Autodesk Fusion 360 part; units mm, degrees
(part 12 of 14)
  line L8266 (240.2049, 412.75) -> (245.7042, 403.225)
  line L8267 (245.7042, 403.225) -> (256.7027, 403.225)
  line L8268 (262.202, 412.75) -> (256.7027, 422.275)
  line L8269 (256.7027, 403.225) -> (262.202, 412.75)
  line L8270 (275.9501, 433.3875) -> (264.9516, 433.3875)
  line L8271 (264.9516, 433.3875) -> (259.4524, 423.8625)
  line L8272 (259.4524, 423.8625) -> (264.9516, 414.3375)
  line L8273 (264.9516, 414.3375) -> (275.9501, 414.3375)
  line L8274 (281.4494, 423.8625) -> (275.9501, 433.3875)
  line L8275 (275.9501, 414.3375) -> (281.4494, 423.8625)
  line L8276 (295.1976, 444.5) -> (284.199, 444.5)
  line L8277 (284.199, 444.5) -> (278.6998, 434.975)
  line L8278 (278.6998, 434.975) -> (284.199, 425.45)
  line L8279 (284.199, 425.45) -> (295.1976, 425.45)
  line L8280 (300.6968, 434.975) -> (295.1976, 444.5)
  line L8281 (295.1976, 425.45) -> (300.6968, 434.975)
  line L8282 (314.445, 455.6125) -> (303.4464, 455.6125)
  line L8283 (303.4464, 455.6125) -> (297.9472, 446.0875)
  line L8284 (297.9472, 446.0875) -> (303.4464, 436.5625)
  line L8285 (303.4464, 436.5625) -> (314.445, 436.5625)
  line L8286 (319.9442, 446.0875) -> (314.445, 455.6125)
  line L8287 (314.445, 436.5625) -> (319.9442, 446.0875)
  line L8288 (333.6924, 466.725) -> (322.6939, 466.725)
  line L8289 (322.6939, 466.725) -> (317.1946, 457.2)
  line L8290 (317.1946, 457.2) -> (322.6939, 447.675)
  line L8291 (322.6939, 447.675) -> (333.6924, 447.675)
  line L8292 (339.1916, 457.2) -> (333.6924, 466.725)
  line L8293 (333.6924, 447.675) -> (339.1916, 457.2)
  line L8294 (-821.1525, -177.8) -> (-832.151, -177.8)
  line L8295 (-832.151, -177.8) -> (-837.6503, -187.325)
  line L8296 (-837.6503, -187.325) -> (-832.151, -196.85)
  line L8297 (-832.151, -196.85) -> (-821.1525, -196.85)
  line L8298 (-815.6532, -187.325) -> (-821.1525, -177.8)
  line L8299 (-821.1525, -196.85) -> (-815.6532, -187.325)
  line L8300 (-801.9051, -166.6875) -> (-812.9036, -166.6875)
  line L8301 (-812.9036, -166.6875) -> (-818.4029, -176.2125)
  line L8302 (-818.4029, -176.2125) -> (-812.9036, -185.7375)
  line L8303 (-812.9036, -185.7375) -> (-801.9051, -185.7375)
  line L8304 (-796.4058, -176.2125) -> (-801.9051, -166.6875)
  line L8305 (-801.9051, -185.7375) -> (-796.4058, -176.2125)
  line L8306 (-782.6577, -155.575) -> (-793.6562, -155.575)
  line L8307 (-793.6562, -155.575) -> (-799.1554, -165.1)
  line L8308 (-799.1554, -165.1) -> (-793.6562, -174.625)
  line L8309 (-793.6562, -174.625) -> (-782.6577, -174.625)
  line L8310 (-777.1584, -165.1) -> (-782.6577, -155.575)
  line L8311 (-782.6577, -174.625) -> (-777.1584, -165.1)
  line L8312 (-763.4102, -144.4625) -> (-774.4088, -144.4625)
  line L8313 (-774.4088, -144.4625) -> (-779.908, -153.9875)
  line L8314 (-779.908, -153.9875) -> (-774.4088, -163.5125)
  line L8315 (-774.4088, -163.5125) -> (-763.4102, -163.5125)
  line L8316 (-757.911, -153.9875) -> (-763.4102, -144.4625)
  line L8317 (-763.4102, -163.5125) -> (-757.911, -153.9875)
  line L8318 (-744.1628, -133.35) -> (-755.1614, -133.35)
  line L8319 (-755.1614, -133.35) -> (-760.6606, -142.875)
  line L8320 (-760.6606, -142.875) -> (-755.1614, -152.4)
  line L8321 (-755.1614, -152.4) -> (-744.1628, -152.4)
  line L8322 (-738.6636, -142.875) -> (-744.1628, -133.35)
  line L8323 (-744.1628, -152.4) -> (-738.6636, -142.875)
  line L8324 (-724.9154, -122.2375) -> (-735.9139, -122.2375)
  line L8325 (-735.9139, -122.2375) -> (-741.4132, -131.7625)
  line L8326 (-741.4132, -131.7625) -> (-735.9139, -141.2875)
  line L8327 (-735.9139, -141.2875) -> (-724.9154, -141.2875)
  line L8328 (-719.4162, -131.7625) -> (-724.9154, -122.2375)
  line L8329 (-724.9154, -141.2875) -> (-719.4162, -131.7625)
  line L8330 (-705.668, -111.125) -> (-716.6665, -111.125)
  line L8331 (-716.6665, -111.125) -> (-722.1658, -120.65)
  line L8332 (-722.1658, -120.65) -> (-716.6665, -130.175)
  line L8333 (-716.6665, -130.175) -> (-705.668, -130.175)
  line L8334 (-700.1687, -120.65) -> (-705.668, -111.125)
  line L8335 (-705.668, -130.175) -> (-700.1687, -120.65)
  line L8336 (-686.4206, -100.0125) -> (-697.4191, -100.0125)
  line L8337 (-697.4191, -100.0125) -> (-702.9184, -109.5375)
  line L8338 (-702.9184, -109.5375) -> (-697.4191, -119.0625)
  line L8339 (-697.4191, -119.0625) -> (-686.4206, -119.0625)
  line L8340 (-680.9213, -109.5375) -> (-686.4206, -100.0125)
  line L8341 (-686.4206, -119.0625) -> (-680.9213, -109.5375)
  line L8342 (-667.1732, -88.9) -> (-678.1717, -88.9)
  line L8343 (-678.1717, -88.9) -> (-683.671, -98.425)
  line L8344 (-683.671, -98.425) -> (-678.1717, -107.95)
  line L8345 (-678.1717, -107.95) -> (-667.1732, -107.95)
  line L8346 (-661.6739, -98.425) -> (-667.1732, -88.9)
  line L8347 (-667.1732, -107.95) -> (-661.6739, -98.425)
  line L8348 (-647.9258, -77.7875) -> (-658.9243, -77.7875)
  line L8349 (-658.9243, -77.7875) -> (-664.4235, -87.3125)
  line L8350 (-664.4235, -87.3125) -> (-658.9243, -96.8375)
  line L8351 (-658.9243, -96.8375) -> (-647.9258, -96.8375)
  line L8352 (-642.4265, -87.3125) -> (-647.9258, -77.7875)
  line L8353 (-647.9258, -96.8375) -> (-642.4265, -87.3125)
  line L8354 (-628.6783, -66.675) -> (-639.6769, -66.675)
  line L8355 (-639.6769, -66.675) -> (-645.1761, -76.2)
  line L8356 (-645.1761, -76.2) -> (-639.6769, -85.725)
  line L8357 (-639.6769, -85.725) -> (-628.6783, -85.725)
  line L8358 (-623.1791, -76.2) -> (-628.6783, -66.675)
  line L8359 (-628.6783, -85.725) -> (-623.1791, -76.2)
  line L8360 (-609.4309, -55.5625) -> (-620.4295, -55.5625)
  line L8361 (-620.4295, -55.5625) -> (-625.9287, -65.0875)
  line L8362 (-625.9287, -65.0875) -> (-620.4295, -74.6125)
  line L8363 (-620.4295, -74.6125) -> (-609.4309, -74.6125)
  line L8364 (-603.9317, -65.0875) -> (-609.4309, -55.5625)
  line L8365 (-609.4309, -74.6125) -> (-603.9317, -65.0875)
  line L8366 (-590.1835, -44.45) -> (-601.182, -44.45)
  line L8367 (-601.182, -44.45) -> (-606.6813, -53.975)
  line L8368 (-606.6813, -53.975) -> (-601.182, -63.5)
  line L8369 (-601.182, -63.5) -> (-590.1835, -63.5)
  line L8370 (-584.6843, -53.975) -> (-590.1835, -44.45)
  line L8371 (-590.1835, -63.5) -> (-584.6843, -53.975)
  line L8372 (-570.9361, -33.3375) -> (-581.9346, -33.3375)
  line L8373 (-581.9346, -33.3375) -> (-587.4339, -42.8625)
  line L8374 (-587.4339, -42.8625) -> (-581.9346, -52.3875)
  line L8375 (-581.9346, -52.3875) -> (-570.9361, -52.3875)
  line L8376 (-565.4368, -42.8625) -> (-570.9361, -33.3375)
  line L8377 (-570.9361, -52.3875) -> (-565.4368, -42.8625)
  line L8378 (-551.6887, -22.225) -> (-562.6872, -22.225)
  line L8379 (-562.6872, -22.225) -> (-568.1865, -31.75)
  line L8380 (-568.1865, -31.75) -> (-562.6872, -41.275)
  line L8381 (-562.6872, -41.275) -> (-551.6887, -41.275)
  line L8382 (-546.1894, -31.75) -> (-551.6887, -22.225)
  line L8383 (-551.6887, -41.275) -> (-546.1894, -31.75)
  line L8384 (-532.4413, -11.1125) -> (-543.4398, -11.1125)
  line L8385 (-543.4398, -11.1125) -> (-548.9391, -20.6375)
  line L8386 (-548.9391, -20.6375) -> (-543.4398, -30.1625)
  line L8387 (-543.4398, -30.1625) -> (-532.4413, -30.1625)
  line L8388 (-526.942, -20.6375) -> (-532.4413, -11.1125)
  line L8389 (-532.4413, -30.1625) -> (-526.942, -20.6375)
  line L8390 (-513.1939, 0) -> (-524.1924, 0)
  line L8391 (-524.1924, 0) -> (-529.6916, -9.525)
  line L8392 (-529.6916, -9.525) -> (-524.1924, -19.05)
  line L8393 (-524.1924, -19.05) -> (-513.1939, -19.05)
  line L8394 (-507.6946, -9.525) -> (-513.1939, 0)
  line L8395 (-513.1939, -19.05) -> (-507.6946, -9.525)
  line L8396 (-493.9464, 11.1125) -> (-504.945, 11.1125)
  line L8397 (-504.945, 11.1125) -> (-510.4442, 1.5875)
  line L8398 (-510.4442, 1.5875) -> (-504.945, -7.9375)
  line L8399 (-504.945, -7.9375) -> (-493.9464, -7.9375)
  line L8400 (-488.4472, 1.5875) -> (-493.9464, 11.1125)
  line L8401 (-493.9464, -7.9375) -> (-488.4472, 1.5875)
  line L8402 (-474.699, 22.225) -> (-485.6976, 22.225)
  line L8403 (-485.6976, 22.225) -> (-491.1968, 12.7)
  line L8404 (-491.1968, 12.7) -> (-485.6976, 3.175)
  line L8405 (-485.6976, 3.175) -> (-474.699, 3.175)
  line L8406 (-469.1998, 12.7) -> (-474.699, 22.225)
  line L8407 (-474.699, 3.175) -> (-469.1998, 12.7)
  line L8408 (-455.4516, 33.3375) -> (-466.4501, 33.3375)
  line L8409 (-466.4501, 33.3375) -> (-471.9494, 23.8125)
  line L8410 (-471.9494, 23.8125) -> (-466.4501, 14.2875)
  line L8411 (-466.4501, 14.2875) -> (-455.4516, 14.2875)
  line L8412 (-449.9524, 23.8125) -> (-455.4516, 33.3375)
  line L8413 (-455.4516, 14.2875) -> (-449.9524, 23.8125)
  line L8414 (-436.2042, 44.45) -> (-447.2027, 44.45)
  line L8415 (-447.2027, 44.45) -> (-452.702, 34.925)
  line L8416 (-452.702, 34.925) -> (-447.2027, 25.4)
  line L8417 (-447.2027, 25.4) -> (-436.2042, 25.4)
  line L8418 (-430.7049, 34.925) -> (-436.2042, 44.45)
  line L8419 (-436.2042, 25.4) -> (-430.7049, 34.925)
  line L8420 (-416.9568, 55.5625) -> (-427.9553, 55.5625)
  line L8421 (-427.9553, 55.5625) -> (-433.4546, 46.0375)
  line L8422 (-433.4546, 46.0375) -> (-427.9553, 36.5125)
  line L8423 (-427.9553, 36.5125) -> (-416.9568, 36.5125)
  line L8424 (-411.4575, 46.0375) -> (-416.9568, 55.5625)
  line L8425 (-416.9568, 36.5125) -> (-411.4575, 46.0375)
  line L8426 (-397.7094, 66.675) -> (-408.7079, 66.675)
  line L8427 (-408.7079, 66.675) -> (-414.2072, 57.15)
  line L8428 (-414.2072, 57.15) -> (-408.7079, 47.625)
  line L8429 (-408.7079, 47.625) -> (-397.7094, 47.625)
  line L8430 (-392.2101, 57.15) -> (-397.7094, 66.675)
  line L8431 (-397.7094, 47.625) -> (-392.2101, 57.15)
  line L8432 (-378.462, 77.7875) -> (-389.4605, 77.7875)
  line L8433 (-389.4605, 77.7875) -> (-394.9597, 68.2625)
  line L8434 (-394.9597, 68.2625) -> (-389.4605, 58.7375)
  line L8435 (-389.4605, 58.7375) -> (-378.462, 58.7375)
  line L8436 (-372.9627, 68.2625) -> (-378.462, 77.7875)
  line L8437 (-378.462, 58.7375) -> (-372.9627, 68.2625)
  line L8438 (-359.2145, 88.9) -> (-370.2131, 88.9)
  line L8439 (-370.2131, 88.9) -> (-375.7123, 79.375)
  line L8440 (-375.7123, 79.375) -> (-370.2131, 69.85)
  line L8441 (-370.2131, 69.85) -> (-359.2145, 69.85)
  line L8442 (-353.7153, 79.375) -> (-359.2145, 88.9)
  line L8443 (-359.2145, 69.85) -> (-353.7153, 79.375)
  line L8444 (-339.9671, 100.0125) -> (-350.9657, 100.0125)
  line L8445 (-350.9657, 100.0125) -> (-356.4649, 90.4875)
  line L8446 (-356.4649, 90.4875) -> (-350.9657, 80.9625)
  line L8447 (-350.9657, 80.9625) -> (-339.9671, 80.9625)
  line L8448 (-334.4679, 90.4875) -> (-339.9671, 100.0125)
  line L8449 (-339.9671, 80.9625) -> (-334.4679, 90.4875)
  line L8450 (-320.7197, 111.125) -> (-331.7182, 111.125)
  line L8451 (-331.7182, 111.125) -> (-337.2175, 101.6)
  line L8452 (-337.2175, 101.6) -> (-331.7182, 92.075)
  line L8453 (-331.7182, 92.075) -> (-320.7197, 92.075)
  line L8454 (-315.2205, 101.6) -> (-320.7197, 111.125)
  line L8455 (-320.7197, 92.075) -> (-315.2205, 101.6)
  line L8456 (-301.4723, 122.2375) -> (-312.4708, 122.2375)
  line L8457 (-312.4708, 122.2375) -> (-317.9701, 112.7125)
  line L8458 (-317.9701, 112.7125) -> (-312.4708, 103.1875)
  line L8459 (-312.4708, 103.1875) -> (-301.4723, 103.1875)
  line L8460 (-295.973, 112.7125) -> (-301.4723, 122.2375)
  line L8461 (-301.4723, 103.1875) -> (-295.973, 112.7125)
  line L8462 (-282.2249, 133.35) -> (-293.2234, 133.35)
  line L8463 (-293.2234, 133.35) -> (-298.7227, 123.825)
  line L8464 (-298.7227, 123.825) -> (-293.2234, 114.3)
  line L8465 (-293.2234, 114.3) -> (-282.2249, 114.3)
  line L8466 (-276.7256, 123.825) -> (-282.2249, 133.35)
  line L8467 (-282.2249, 114.3) -> (-276.7256, 123.825)
  line L8468 (-262.9775, 144.4625) -> (-273.976, 144.4625)
  line L8469 (-273.976, 144.4625) -> (-279.4753, 134.9375)
  line L8470 (-279.4753, 134.9375) -> (-273.976, 125.4125)
  line L8471 (-273.976, 125.4125) -> (-262.9775, 125.4125)
  line L8472 (-257.4782, 134.9375) -> (-262.9775, 144.4625)
  line L8473 (-262.9775, 125.4125) -> (-257.4782, 134.9375)
  line L8474 (-243.7301, 155.575) -> (-254.7286, 155.575)
  line L8475 (-254.7286, 155.575) -> (-260.2278, 146.05)
  line L8476 (-260.2278, 146.05) -> (-254.7286, 136.525)
  line L8477 (-254.7286, 136.525) -> (-243.7301, 136.525)
  line L8478 (-238.2308, 146.05) -> (-243.7301, 155.575)
  line L8479 (-243.7301, 136.525) -> (-238.2308, 146.05)
  line L8480 (-224.4826, 166.6875) -> (-235.4812, 166.6875)
  line L8481 (-235.4812, 166.6875) -> (-240.9804, 157.1625)
  line L8482 (-240.9804, 157.1625) -> (-235.4812, 147.6375)
  line L8483 (-235.4812, 147.6375) -> (-224.4826, 147.6375)
  line L8484 (-218.9834, 157.1625) -> (-224.4826, 166.6875)
  line L8485 (-224.4826, 147.6375) -> (-218.9834, 157.1625)
  line L8486 (-205.2352, 177.8) -> (-216.2337, 177.8)
  line L8487 (-216.2337, 177.8) -> (-221.733, 168.275)
  line L8488 (-221.733, 168.275) -> (-216.2337, 158.75)
  line L8489 (-216.2337, 158.75) -> (-205.2352, 158.75)
  line L8490 (-199.736, 168.275) -> (-205.2352, 177.8)
  line L8491 (-205.2352, 158.75) -> (-199.736, 168.275)
  line L8492 (-185.9878, 188.9125) -> (-196.9863, 188.9125)
  line L8493 (-196.9863, 188.9125) -> (-202.4856, 179.3875)
  line L8494 (-202.4856, 179.3875) -> (-196.9863, 169.8625)
  line L8495 (-196.9863, 169.8625) -> (-185.9878, 169.8625)
  line L8496 (-180.4886, 179.3875) -> (-185.9878, 188.9125)
  line L8497 (-185.9878, 169.8625) -> (-180.4886, 179.3875)
  line L8498 (-166.7404, 200.025) -> (-177.7389, 200.025)
  line L8499 (-177.7389, 200.025) -> (-183.2382, 190.5)
  line L8500 (-183.2382, 190.5) -> (-177.7389, 180.975)
  line L8501 (-177.7389, 180.975) -> (-166.7404, 180.975)
  line L8502 (-161.2411, 190.5) -> (-166.7404, 200.025)
  line L8503 (-166.7404, 180.975) -> (-161.2411, 190.5)
  line L8504 (-147.493, 211.1375) -> (-158.4915, 211.1375)
  line L8505 (-158.4915, 211.1375) -> (-163.9908, 201.6125)
  line L8506 (-163.9908, 201.6125) -> (-158.4915, 192.0875)
  line L8507 (-158.4915, 192.0875) -> (-147.493, 192.0875)
  line L8508 (-141.9937, 201.6125) -> (-147.493, 211.1375)
  line L8509 (-147.493, 192.0875) -> (-141.9937, 201.6125)
  line L8510 (-128.2456, 222.25) -> (-139.2441, 222.25)
  line L8511 (-139.2441, 222.25) -> (-144.7434, 212.725)
  line L8512 (-144.7434, 212.725) -> (-139.2441, 203.2)
  line L8513 (-139.2441, 203.2) -> (-128.2456, 203.2)
  line L8514 (-122.7463, 212.725) -> (-128.2456, 222.25)
  line L8515 (-128.2456, 203.2) -> (-122.7463, 212.725)
  line L8516 (-108.9982, 233.3625) -> (-119.9967, 233.3625)
  line L8517 (-119.9967, 233.3625) -> (-125.4959, 223.8375)
  line L8518 (-125.4959, 223.8375) -> (-119.9967, 214.3125)
  line L8519 (-119.9967, 214.3125) -> (-108.9982, 214.3125)
  line L8520 (-103.4989, 223.8375) -> (-108.9982, 233.3625)
  line L8521 (-108.9982, 214.3125) -> (-103.4989, 223.8375)
  line L8522 (-89.7507, 244.475) -> (-100.7493, 244.475)
  line L8523 (-100.7493, 244.475) -> (-106.2485, 234.95)
  line L8524 (-106.2485, 234.95) -> (-100.7493, 225.425)
  line L8525 (-100.7493, 225.425) -> (-89.7507, 225.425)
  line L8526 (-84.2515, 234.95) -> (-89.7507, 244.475)
  line L8527 (-89.7507, 225.425) -> (-84.2515, 234.95)
  line L8528 (-70.5033, 255.5875) -> (-81.5018, 255.5875)
  line L8529 (-81.5018, 255.5875) -> (-87.0011, 246.0625)
  line L8530 (-87.0011, 246.0625) -> (-81.5018, 236.5375)
  line L8531 (-81.5018, 236.5375) -> (-70.5033, 236.5375)
  line L8532 (-65.0041, 246.0625) -> (-70.5033, 255.5875)
  line L8533 (-70.5033, 236.5375) -> (-65.0041, 246.0625)
  line L8534 (-51.2559, 266.7) -> (-62.2544, 266.7)
  line L8535 (-62.2544, 266.7) -> (-67.7537, 257.175)
  line L8536 (-67.7537, 257.175) -> (-62.2544, 247.65)
  line L8537 (-62.2544, 247.65) -> (-51.2559, 247.65)
  line L8538 (-45.7566, 257.175) -> (-51.2559, 266.7)
  line L8539 (-51.2559, 247.65) -> (-45.7566, 257.175)
  line L8540 (-32.0085, 277.8125) -> (-43.007, 277.8125)
  line L8541 (-43.007, 277.8125) -> (-48.5063, 268.2875)
  line L8542 (-48.5063, 268.2875) -> (-43.007, 258.7625)
  line L8543 (-43.007, 258.7625) -> (-32.0085, 258.7625)
  line L8544 (-26.5092, 268.2875) -> (-32.0085, 277.8125)
  line L8545 (-32.0085, 258.7625) -> (-26.5092, 268.2875)
  line L8546 (-12.7611, 288.925) -> (-23.7596, 288.925)
  line L8547 (-23.7596, 288.925) -> (-29.2589, 279.4)
  line L8548 (-29.2589, 279.4) -> (-23.7596, 269.875)
  line L8549 (-23.7596, 269.875) -> (-12.7611, 269.875)
  line L8550 (-7.2618, 279.4) -> (-12.7611, 288.925)
  line L8551 (-12.7611, 269.875) -> (-7.2618, 279.4)
  line L8552 (6.4863, 300.0375) -> (-4.5122, 300.0375)
  line L8553 (-4.5122, 300.0375) -> (-10.0114, 290.5125)
  line L8554 (-10.0114, 290.5125) -> (-4.5122, 280.9875)
  line L8555 (-4.5122, 280.9875) -> (6.4863, 280.9875)
  line L8556 (11.9856, 290.5125) -> (6.4863, 300.0375)
  line L8557 (6.4863, 280.9875) -> (11.9856, 290.5125)
  line L8558 (25.7337, 311.15) -> (14.7352, 311.15)
  line L8559 (14.7352, 311.15) -> (9.236, 301.625)
  line L8560 (9.236, 301.625) -> (14.7352, 292.1)
  line L8561 (14.7352, 292.1) -> (25.7337, 292.1)
  line L8562 (31.233, 301.625) -> (25.7337, 311.15)
  line L8563 (25.7337, 292.1) -> (31.233, 301.625)
  line L8564 (44.9812, 322.2625) -> (33.9826, 322.2625)
  line L8565 (33.9826, 322.2625) -> (28.4834, 312.7375)
  line L8566 (28.4834, 312.7375) -> (33.9826, 303.2125)
  line L8567 (33.9826, 303.2125) -> (44.9812, 303.2125)
  line L8568 (50.4804, 312.7375) -> (44.9812, 322.2625)
  line L8569 (44.9812, 303.2125) -> (50.4804, 312.7375)
  line L8570 (64.2286, 333.375) -> (53.2301, 333.375)
  line L8571 (53.2301, 333.375) -> (47.7308, 323.85)
  line L8572 (47.7308, 323.85) -> (53.2301, 314.325)
  line L8573 (53.2301, 314.325) -> (64.2286, 314.325)
  line L8574 (69.7278, 323.85) -> (64.2286, 333.375)
  line L8575 (64.2286, 314.325) -> (69.7278, 323.85)
  line L8576 (83.476, 344.4875) -> (72.4775, 344.4875)
  line L8577 (72.4775, 344.4875) -> (66.9782, 334.9625)
  line L8578 (66.9782, 334.9625) -> (72.4775, 325.4375)
  line L8579 (72.4775, 325.4375) -> (83.476, 325.4375)
  line L8580 (88.9753, 334.9625) -> (83.476, 344.4875)
  line L8581 (83.476, 325.4375) -> (88.9753, 334.9625)
  line L8582 (102.7234, 355.6) -> (91.7249, 355.6)
  line L8583 (91.7249, 355.6) -> (86.2256, 346.075)
  line L8584 (86.2256, 346.075) -> (91.7249, 336.55)
  line L8585 (91.7249, 336.55) -> (102.7234, 336.55)
  line L8586 (108.2227, 346.075) -> (102.7234, 355.6)
  line L8587 (102.7234, 336.55) -> (108.2227, 346.075)
  line L8588 (121.9708, 366.7125) -> (110.9723, 366.7125)
  line L8589 (110.9723, 366.7125) -> (105.473, 357.1875)
  line L8590 (105.473, 357.1875) -> (110.9723, 347.6625)
  line L8591 (110.9723, 347.6625) -> (121.9708, 347.6625)
  line L8592 (127.4701, 357.1875) -> (121.9708, 366.7125)
  line L8593 (121.9708, 347.6625) -> (127.4701, 357.1875)
  line L8594 (141.2182, 377.825) -> (130.2197, 377.825)
  line L8595 (130.2197, 377.825) -> (124.7205, 368.3)
  line L8596 (124.7205, 368.3) -> (130.2197, 358.775)
  line L8597 (130.2197, 358.775) -> (141.2182, 358.775)
  line L8598 (146.7175, 368.3) -> (141.2182, 377.825)
  line L8599 (141.2182, 358.775) -> (146.7175, 368.3)
  line L8600 (160.4657, 388.9375) -> (149.4671, 388.9375)
  line L8601 (149.4671, 388.9375) -> (143.9679, 379.4125)
  line L8602 (143.9679, 379.4125) -> (149.4671, 369.8875)
  line L8603 (149.4671, 369.8875) -> (160.4657, 369.8875)
  line L8604 (165.9649, 379.4125) -> (160.4657, 388.9375)
  line L8605 (160.4657, 369.8875) -> (165.9649, 379.4125)
  line L8606 (179.7131, 400.05) -> (168.7145, 400.05)
  line L8607 (168.7145, 400.05) -> (163.2153, 390.525)
  line L8608 (163.2153, 390.525) -> (168.7145, 381)
  line L8609 (168.7145, 381) -> (179.7131, 381)
  line L8610 (185.2123, 390.525) -> (179.7131, 400.05)
  line L8611 (179.7131, 381) -> (185.2123, 390.525)
  line L8612 (198.9605, 411.1625) -> (187.962, 411.1625)
  line L8613 (187.962, 411.1625) -> (182.4627, 401.6375)
  line L8614 (182.4627, 401.6375) -> (187.962, 392.1125)
  line L8615 (187.962, 392.1125) -> (198.9605, 392.1125)
  line L8616 (204.4597, 401.6375) -> (198.9605, 411.1625)
  line L8617 (198.9605, 392.1125) -> (204.4597, 401.6375)
  line L8618 (218.2079, 422.275) -> (207.2094, 422.275)
  line L8619 (207.2094, 422.275) -> (201.7101, 412.75)
  line L8620 (201.7101, 412.75) -> (207.2094, 403.225)
  line L8621 (207.2094, 403.225) -> (218.2079, 403.225)
  line L8622 (223.7072, 412.75) -> (218.2079, 422.275)
  line L8623 (218.2079, 403.225) -> (223.7072, 412.75)
  line L8624 (237.4553, 433.3875) -> (226.4568, 433.3875)
  line L8625 (226.4568, 433.3875) -> (220.9575, 423.8625)
  line L8626 (220.9575, 423.8625) -> (226.4568, 414.3375)
  line L8627 (226.4568, 414.3375) -> (237.4553, 414.3375)
  line L8628 (242.9546, 423.8625) -> (237.4553, 433.3875)
  line L8629 (237.4553, 414.3375) -> (242.9546, 423.8625)
  line L8630 (256.7027, 444.5) -> (245.7042, 444.5)
  line L8631 (245.7042, 444.5) -> (240.2049, 434.975)
  line L8632 (240.2049, 434.975) -> (245.7042, 425.45)
  line L8633 (245.7042, 425.45) -> (256.7027, 425.45)
  line L8634 (262.202, 434.975) -> (256.7027, 444.5)
  line L8635 (256.7027, 425.45) -> (262.202, 434.975)
  line L8636 (275.9501, 455.6125) -> (264.9516, 455.6125)
  line L8637 (264.9516, 455.6125) -> (259.4524, 446.0875)
  line L8638 (259.4524, 446.0875) -> (264.9516, 436.5625)
  line L8639 (264.9516, 436.5625) -> (275.9501, 436.5625)
  line L8640 (281.4494, 446.0875) -> (275.9501, 455.6125)
  line L8641 (275.9501, 436.5625) -> (281.4494, 446.0875)
  line L8642 (295.1976, 466.725) -> (284.199, 466.725)
  line L8643 (284.199, 466.725) -> (278.6998, 457.2)
  line L8644 (278.6998, 457.2) -> (284.199, 447.675)
  line L8645 (284.199, 447.675) -> (295.1976, 447.675)
  line L8646 (300.6968, 457.2) -> (295.1976, 466.725)
  line L8647 (295.1976, 447.675) -> (300.6968, 457.2)
  line L8648 (314.445, 477.8375) -> (303.4464, 477.8375)
  line L8649 (303.4464, 477.8375) -> (297.9472, 468.3125)
  line L8650 (297.9472, 468.3125) -> (303.4464, 458.7875)
  line L8651 (303.4464, 458.7875) -> (314.445, 458.7875)
  line L8652 (319.9442, 468.3125) -> (314.445, 477.8375)
  line L8653 (314.445, 458.7875) -> (319.9442, 468.3125)
  line L8654 (-840.3999, -166.6875) -> (-851.3984, -166.6875)
  line L8655 (-851.3984, -166.6875) -> (-856.8977, -176.2125)
  line L8656 (-856.8977, -176.2125) -> (-851.3984, -185.7375)
  line L8657 (-851.3984, -185.7375) -> (-840.3999, -185.7375)
  line L8658 (-834.9006, -176.2125) -> (-840.3999, -166.6875)
  line L8659 (-840.3999, -185.7375) -> (-834.9006, -176.2125)
  line L8660 (-821.1525, -155.575) -> (-832.151, -155.575)
  line L8661 (-832.151, -155.575) -> (-837.6503, -165.1)
  line L8662 (-837.6503, -165.1) -> (-832.151, -174.625)
  line L8663 (-832.151, -174.625) -> (-821.1525, -174.625)
  line L8664 (-815.6532, -165.1) -> (-821.1525, -155.575)
  line L8665 (-821.1525, -174.625) -> (-815.6532, -165.1)
  line L8666 (-801.9051, -144.4625) -> (-812.9036, -144.4625)
  line L8667 (-812.9036, -144.4625) -> (-818.4029, -153.9875)
  line L8668 (-818.4029, -153.9875) -> (-812.9036, -163.5125)
  line L8669 (-812.9036, -163.5125) -> (-801.9051, -163.5125)
  line L8670 (-796.4058, -153.9875) -> (-801.9051, -144.4625)
  line L8671 (-801.9051, -163.5125) -> (-796.4058, -153.9875)
  line L8672 (-782.6577, -133.35) -> (-793.6562, -133.35)
  line L8673 (-793.6562, -133.35) -> (-799.1554, -142.875)
  line L8674 (-799.1554, -142.875) -> (-793.6562, -152.4)
  line L8675 (-793.6562, -152.4) -> (-782.6577, -152.4)
  line L8676 (-777.1584, -142.875) -> (-782.6577, -133.35)
  line L8677 (-782.6577, -152.4) -> (-777.1584, -142.875)
  line L8678 (-763.4102, -122.2375) -> (-774.4088, -122.2375)
  line L8679 (-774.4088, -122.2375) -> (-779.908, -131.7625)
  line L8680 (-779.908, -131.7625) -> (-774.4088, -141.2875)
  line L8681 (-774.4088, -141.2875) -> (-763.4102, -141.2875)
  line L8682 (-757.911, -131.7625) -> (-763.4102, -122.2375)
  line L8683 (-763.4102, -141.2875) -> (-757.911, -131.7625)
  line L8684 (-744.1628, -111.125) -> (-755.1614, -111.125)
  line L8685 (-755.1614, -111.125) -> (-760.6606, -120.65)
  line L8686 (-760.6606, -120.65) -> (-755.1614, -130.175)
  line L8687 (-755.1614, -130.175) -> (-744.1628, -130.175)
  line L8688 (-738.6636, -120.65) -> (-744.1628, -111.125)
  line L8689 (-744.1628, -130.175) -> (-738.6636, -120.65)
  line L8690 (-724.9154, -100.0125) -> (-735.9139, -100.0125)
  line L8691 (-735.9139, -100.0125) -> (-741.4132, -109.5375)
  line L8692 (-741.4132, -109.5375) -> (-735.9139, -119.0625)
  line L8693 (-735.9139, -119.0625) -> (-724.9154, -119.0625)
  line L8694 (-719.4162, -109.5375) -> (-724.9154, -100.0125)
  line L8695 (-724.9154, -119.0625) -> (-719.4162, -109.5375)
  line L8696 (-705.668, -88.9) -> (-716.6665, -88.9)
  line L8697 (-716.6665, -88.9) -> (-722.1658, -98.425)
  line L8698 (-722.1658, -98.425) -> (-716.6665, -107.95)
  line L8699 (-716.6665, -107.95) -> (-705.668, -107.95)
  line L8700 (-700.1687, -98.425) -> (-705.668, -88.9)
  line L8701 (-705.668, -107.95) -> (-700.1687, -98.425)
  line L8702 (-686.4206, -77.7875) -> (-697.4191, -77.7875)
  line L8703 (-697.4191, -77.7875) -> (-702.9184, -87.3125)
  line L8704 (-702.9184, -87.3125) -> (-697.4191, -96.8375)
  line L8705 (-697.4191, -96.8375) -> (-686.4206, -96.8375)
  line L8706 (-680.9213, -87.3125) -> (-686.4206, -77.7875)
  line L8707 (-686.4206, -96.8375) -> (-680.9213, -87.3125)
  line L8708 (-667.1732, -66.675) -> (-678.1717, -66.675)
  line L8709 (-678.1717, -66.675) -> (-683.671, -76.2)
  line L8710 (-683.671, -76.2) -> (-678.1717, -85.725)
  line L8711 (-678.1717, -85.725) -> (-667.1732, -85.725)
  line L8712 (-661.6739, -76.2) -> (-667.1732, -66.675)
  line L8713 (-667.1732, -85.725) -> (-661.6739, -76.2)
  line L8714 (-647.9258, -55.5625) -> (-658.9243, -55.5625)
  line L8715 (-658.9243, -55.5625) -> (-664.4235, -65.0875)
  line L8716 (-664.4235, -65.0875) -> (-658.9243, -74.6125)
  line L8717 (-658.9243, -74.6125) -> (-647.9258, -74.6125)
  line L8718 (-642.4265, -65.0875) -> (-647.9258, -55.5625)
  line L8719 (-647.9258, -74.6125) -> (-642.4265, -65.0875)
  line L8720 (-628.6783, -44.45) -> (-639.6769, -44.45)
  line L8721 (-639.6769, -44.45) -> (-645.1761, -53.975)
  line L8722 (-645.1761, -53.975) -> (-639.6769, -63.5)
  line L8723 (-639.6769, -63.5) -> (-628.6783, -63.5)
  line L8724 (-623.1791, -53.975) -> (-628.6783, -44.45)
  line L8725 (-628.6783, -63.5) -> (-623.1791, -53.975)
  line L8726 (-609.4309, -33.3375) -> (-620.4295, -33.3375)
  line L8727 (-620.4295, -33.3375) -> (-625.9287, -42.8625)
  line L8728 (-625.9287, -42.8625) -> (-620.4295, -52.3875)
  line L8729 (-620.4295, -52.3875) -> (-609.4309, -52.3875)
  line L8730 (-603.9317, -42.8625) -> (-609.4309, -33.3375)
  line L8731 (-609.4309, -52.3875) -> (-603.9317, -42.8625)
  line L8732 (-590.1835, -22.225) -> (-601.182, -22.225)
  line L8733 (-601.182, -22.225) -> (-606.6813, -31.75)
  line L8734 (-606.6813, -31.75) -> (-601.182, -41.275)
  line L8735 (-601.182, -41.275) -> (-590.1835, -41.275)
  line L8736 (-584.6843, -31.75) -> (-590.1835, -22.225)
  line L8737 (-590.1835, -41.275) -> (-584.6843, -31.75)
  line L8738 (-570.9361, -11.1125) -> (-581.9346, -11.1125)
  line L8739 (-581.9346, -11.1125) -> (-587.4339, -20.6375)
  line L8740 (-587.4339, -20.6375) -> (-581.9346, -30.1625)
  line L8741 (-581.9346, -30.1625) -> (-570.9361, -30.1625)
  line L8742 (-565.4368, -20.6375) -> (-570.9361, -11.1125)
  line L8743 (-570.9361, -30.1625) -> (-565.4368, -20.6375)
  line L8744 (-551.6887, 0) -> (-562.6872, 0)
  line L8745 (-562.6872, 0) -> (-568.1865, -9.525)
  line L8746 (-568.1865, -9.525) -> (-562.6872, -19.05)
  line L8747 (-562.6872, -19.05) -> (-551.6887, -19.05)
  line L8748 (-546.1894, -9.525) -> (-551.6887, 0)
  line L8749 (-551.6887, -19.05) -> (-546.1894, -9.525)
  line L8750 (-532.4413, 11.1125) -> (-543.4398, 11.1125)
  line L8751 (-543.4398, 11.1125) -> (-548.9391, 1.5875)
  line L8752 (-548.9391, 1.5875) -> (-543.4398, -7.9375)
  line L8753 (-543.4398, -7.9375) -> (-532.4413, -7.9375)
  line L8754 (-526.942, 1.5875) -> (-532.4413, 11.1125)
  line L8755 (-532.4413, -7.9375) -> (-526.942, 1.5875)
  line L8756 (-513.1939, 22.225) -> (-524.1924, 22.225)
  line L8757 (-524.1924, 22.225) -> (-529.6916, 12.7)
  line L8758 (-529.6916, 12.7) -> (-524.1924, 3.175)
  line L8759 (-524.1924, 3.175) -> (-513.1939, 3.175)
  line L8760 (-507.6946, 12.7) -> (-513.1939, 22.225)
  line L8761 (-513.1939, 3.175) -> (-507.6946, 12.7)
  line L8762 (-493.9464, 33.3375) -> (-504.945, 33.3375)
  line L8763 (-504.945, 33.3375) -> (-510.4442, 23.8125)
  line L8764 (-510.4442, 23.8125) -> (-504.945, 14.2875)
  line L8765 (-504.945, 14.2875) -> (-493.9464, 14.2875)
  line L8766 (-488.4472, 23.8125) -> (-493.9464, 33.3375)
  line L8767 (-493.9464, 14.2875) -> (-488.4472, 23.8125)
  line L8768 (-474.699, 44.45) -> (-485.6976, 44.45)
  line L8769 (-485.6976, 44.45) -> (-491.1968, 34.925)
  line L8770 (-491.1968, 34.925) -> (-485.6976, 25.4)
  line L8771 (-485.6976, 25.4) -> (-474.699, 25.4)
  line L8772 (-469.1998, 34.925) -> (-474.699, 44.45)
  line L8773 (-474.699, 25.4) -> (-469.1998, 34.925)
  line L8774 (-455.4516, 55.5625) -> (-466.4501, 55.5625)
  line L8775 (-466.4501, 55.5625) -> (-471.9494, 46.0375)
  line L8776 (-471.9494, 46.0375) -> (-466.4501, 36.5125)
  line L8777 (-466.4501, 36.5125) -> (-455.4516, 36.5125)
  line L8778 (-449.9524, 46.0375) -> (-455.4516, 55.5625)
  line L8779 (-455.4516, 36.5125) -> (-449.9524, 46.0375)
  line L8780 (-436.2042, 66.675) -> (-447.2027, 66.675)
  line L8781 (-447.2027, 66.675) -> (-452.702, 57.15)
  line L8782 (-452.702, 57.15) -> (-447.2027, 47.625)
  line L8783 (-447.2027, 47.625) -> (-436.2042, 47.625)
  line L8784 (-430.7049, 57.15) -> (-436.2042, 66.675)
  line L8785 (-436.2042, 47.625) -> (-430.7049, 57.15)
  line L8786 (-416.9568, 77.7875) -> (-427.9553, 77.7875)
  line L8787 (-427.9553, 77.7875) -> (-433.4546, 68.2625)
  line L8788 (-433.4546, 68.2625) -> (-427.9553, 58.7375)
  line L8789 (-427.9553, 58.7375) -> (-416.9568, 58.7375)
  line L8790 (-411.4575, 68.2625) -> (-416.9568, 77.7875)
  line L8791 (-416.9568, 58.7375) -> (-411.4575, 68.2625)
  line L8792 (-397.7094, 88.9) -> (-408.7079, 88.9)
  line L8793 (-408.7079, 88.9) -> (-414.2072, 79.375)
  line L8794 (-414.2072, 79.375) -> (-408.7079, 69.85)
  line L8795 (-408.7079, 69.85) -> (-397.7094, 69.85)
  line L8796 (-392.2101, 79.375) -> (-397.7094, 88.9)
  line L8797 (-397.7094, 69.85) -> (-392.2101, 79.375)
  line L8798 (-378.462, 100.0125) -> (-389.4605, 100.0125)
  line L8799 (-389.4605, 100.0125) -> (-394.9597, 90.4875)
  line L8800 (-394.9597, 90.4875) -> (-389.4605, 80.9625)
  line L8801 (-389.4605, 80.9625) -> (-378.462, 80.9625)
  line L8802 (-372.9627, 90.4875) -> (-378.462, 100.0125)
  line L8803 (-378.462, 80.9625) -> (-372.9627, 90.4875)
  line L8804 (-359.2145, 111.125) -> (-370.2131, 111.125)
  line L8805 (-370.2131, 111.125) -> (-375.7123, 101.6)
  line L8806 (-375.7123, 101.6) -> (-370.2131, 92.075)
  line L8807 (-370.2131, 92.075) -> (-359.2145, 92.075)
  line L8808 (-353.7153, 101.6) -> (-359.2145, 111.125)
  line L8809 (-359.2145, 92.075) -> (-353.7153, 101.6)
  line L8810 (-339.9671, 122.2375) -> (-350.9657, 122.2375)
  line L8811 (-350.9657, 122.2375) -> (-356.4649, 112.7125)
  line L8812 (-356.4649, 112.7125) -> (-350.9657, 103.1875)
  line L8813 (-350.9657, 103.1875) -> (-339.9671, 103.1875)
  line L8814 (-334.4679, 112.7125) -> (-339.9671, 122.2375)
  line L8815 (-339.9671, 103.1875) -> (-334.4679, 112.7125)
  line L8816 (-320.7197, 133.35) -> (-331.7182, 133.35)
  line L8817 (-331.7182, 133.35) -> (-337.2175, 123.825)
  line L8818 (-337.2175, 123.825) -> (-331.7182, 114.3)
  line L8819 (-331.7182, 114.3) -> (-320.7197, 114.3)
  line L8820 (-315.2205, 123.825) -> (-320.7197, 133.35)
  line L8821 (-320.7197, 114.3) -> (-315.2205, 123.825)
  line L8822 (-301.4723, 144.4625) -> (-312.4708, 144.4625)
  line L8823 (-312.4708, 144.4625) -> (-317.9701, 134.9375)
  line L8824 (-317.9701, 134.9375) -> (-312.4708, 125.4125)
  line L8825 (-312.4708, 125.4125) -> (-301.4723, 125.4125)
  line L8826 (-295.973, 134.9375) -> (-301.4723, 144.4625)
  line L8827 (-301.4723, 125.4125) -> (-295.973, 134.9375)
  line L8828 (-282.2249, 155.575) -> (-293.2234, 155.575)
  line L8829 (-293.2234, 155.575) -> (-298.7227, 146.05)
  line L8830 (-298.7227, 146.05) -> (-293.2234, 136.525)
  line L8831 (-293.2234, 136.525) -> (-282.2249, 136.525)
  line L8832 (-276.7256, 146.05) -> (-282.2249, 155.575)
  line L8833 (-282.2249, 136.525) -> (-276.7256, 146.05)
  line L8834 (-262.9775, 166.6875) -> (-273.976, 166.6875)
  line L8835 (-273.976, 166.6875) -> (-279.4753, 157.1625)
  line L8836 (-279.4753, 157.1625) -> (-273.976, 147.6375)
  line L8837 (-273.976, 147.6375) -> (-262.9775, 147.6375)
  line L8838 (-257.4782, 157.1625) -> (-262.9775, 166.6875)
  line L8839 (-262.9775, 147.6375) -> (-257.4782, 157.1625)
  line L8840 (-243.7301, 177.8) -> (-254.7286, 177.8)
  line L8841 (-254.7286, 177.8) -> (-260.2278, 168.275)
  line L8842 (-260.2278, 168.275) -> (-254.7286, 158.75)
  line L8843 (-254.7286, 158.75) -> (-243.7301, 158.75)
  line L8844 (-238.2308, 168.275) -> (-243.7301, 177.8)
  line L8845 (-243.7301, 158.75) -> (-238.2308, 168.275)
  line L8846 (-224.4826, 188.9125) -> (-235.4812, 188.9125)
  line L8847 (-235.4812, 188.9125) -> (-240.9804, 179.3875)
  line L8848 (-240.9804, 179.3875) -> (-235.4812, 169.8625)
  line L8849 (-235.4812, 169.8625) -> (-224.4826, 169.8625)
  line L8850 (-218.9834, 179.3875) -> (-224.4826, 188.9125)
  line L8851 (-224.4826, 169.8625) -> (-218.9834, 179.3875)
  line L8852 (-205.2352, 200.025) -> (-216.2337, 200.025)
  line L8853 (-216.2337, 200.025) -> (-221.733, 190.5)
  line L8854 (-221.733, 190.5) -> (-216.2337, 180.975)
  line L8855 (-216.2337, 180.975) -> (-205.2352, 180.975)
  line L8856 (-199.736, 190.5) -> (-205.2352, 200.025)
  line L8857 (-205.2352, 180.975) -> (-199.736, 190.5)
  line L8858 (-185.9878, 211.1375) -> (-196.9863, 211.1375)
  line L8859 (-196.9863, 211.1375) -> (-202.4856, 201.6125)
  line L8860 (-202.4856, 201.6125) -> (-196.9863, 192.0875)
  line L8861 (-196.9863, 192.0875) -> (-185.9878, 192.0875)
  line L8862 (-180.4886, 201.6125) -> (-185.9878, 211.1375)
  line L8863 (-185.9878, 192.0875) -> (-180.4886, 201.6125)
  line L8864 (-166.7404, 222.25) -> (-177.7389, 222.25)
  line L8865 (-177.7389, 222.25) -> (-183.2382, 212.725)
  line L8866 (-183.2382, 212.725) -> (-177.7389, 203.2)
  line L8867 (-177.7389, 203.2) -> (-166.7404, 203.2)
  line L8868 (-161.2411, 212.725) -> (-166.7404, 222.25)
  line L8869 (-166.7404, 203.2) -> (-161.2411, 212.725)
  line L8870 (-147.493, 233.3625) -> (-158.4915, 233.3625)
  line L8871 (-158.4915, 233.3625) -> (-163.9908, 223.8375)
  line L8872 (-163.9908, 223.8375) -> (-158.4915, 214.3125)
  line L8873 (-158.4915, 214.3125) -> (-147.493, 214.3125)
  line L8874 (-141.9937, 223.8375) -> (-147.493, 233.3625)
  line L8875 (-147.493, 214.3125) -> (-141.9937, 223.8375)
  line L8876 (-128.2456, 244.475) -> (-139.2441, 244.475)
  line L8877 (-139.2441, 244.475) -> (-144.7434, 234.95)
  line L8878 (-144.7434, 234.95) -> (-139.2441, 225.425)
  line L8879 (-139.2441, 225.425) -> (-128.2456, 225.425)
  line L8880 (-122.7463, 234.95) -> (-128.2456, 244.475)
  line L8881 (-128.2456, 225.425) -> (-122.7463, 234.95)
  line L8882 (-108.9982, 255.5875) -> (-119.9967, 255.5875)
  line L8883 (-119.9967, 255.5875) -> (-125.4959, 246.0625)
  line L8884 (-125.4959, 246.0625) -> (-119.9967, 236.5375)
  line L8885 (-119.9967, 236.5375) -> (-108.9982, 236.5375)
  line L8886 (-103.4989, 246.0625) -> (-108.9982, 255.5875)
  line L8887 (-108.9982, 236.5375) -> (-103.4989, 246.0625)
  line L8888 (-89.7507, 266.7) -> (-100.7493, 266.7)
  line L8889 (-100.7493, 266.7) -> (-106.2485, 257.175)
  line L8890 (-106.2485, 257.175) -> (-100.7493, 247.65)
  line L8891 (-100.7493, 247.65) -> (-89.7507, 247.65)
  line L8892 (-84.2515, 257.175) -> (-89.7507, 266.7)
  line L8893 (-89.7507, 247.65) -> (-84.2515, 257.175)
  line L8894 (-70.5033, 277.8125) -> (-81.5018, 277.8125)
  line L8895 (-81.5018, 277.8125) -> (-87.0011, 268.2875)
  line L8896 (-87.0011, 268.2875) -> (-81.5018, 258.7625)
  line L8897 (-81.5018, 258.7625) -> (-70.5033, 258.7625)
  line L8898 (-65.0041, 268.2875) -> (-70.5033, 277.8125)
  line L8899 (-70.5033, 258.7625) -> (-65.0041, 268.2875)
  line L8900 (-51.2559, 288.925) -> (-62.2544, 288.925)
  line L8901 (-62.2544, 288.925) -> (-67.7537, 279.4)
  line L8902 (-67.7537, 279.4) -> (-62.2544, 269.875)
  line L8903 (-62.2544, 269.875) -> (-51.2559, 269.875)
  line L8904 (-45.7566, 279.4) -> (-51.2559, 288.925)
  line L8905 (-51.2559, 269.875) -> (-45.7566, 279.4)
  line L8906 (-32.0085, 300.0375) -> (-43.007, 300.0375)
  line L8907 (-43.007, 300.0375) -> (-48.5063, 290.5125)
  line L8908 (-48.5063, 290.5125) -> (-43.007, 280.9875)
  line L8909 (-43.007, 280.9875) -> (-32.0085, 280.9875)
  line L8910 (-26.5092, 290.5125) -> (-32.0085, 300.0375)
  line L8911 (-32.0085, 280.9875) -> (-26.5092, 290.5125)
  line L8912 (-12.7611, 311.15) -> (-23.7596, 311.15)
  line L8913 (-23.7596, 311.15) -> (-29.2589, 301.625)
  line L8914 (-29.2589, 301.625) -> (-23.7596, 292.1)
  line L8915 (-23.7596, 292.1) -> (-12.7611, 292.1)
  line L8916 (-7.2618, 301.625) -> (-12.7611, 311.15)
  line L8917 (-12.7611, 292.1) -> (-7.2618, 301.625)
  line L8918 (6.4863, 322.2625) -> (-4.5122, 322.2625)
  line L8919 (-4.5122, 322.2625) -> (-10.0114, 312.7375)
  line L8920 (-10.0114, 312.7375) -> (-4.5122, 303.2125)
  line L8921 (-4.5122, 303.2125) -> (6.4863, 303.2125)
  line L8922 (11.9856, 312.7375) -> (6.4863, 322.2625)
  line L8923 (6.4863, 303.2125) -> (11.9856, 312.7375)
  line L8924 (25.7337, 333.375) -> (14.7352, 333.375)
  line L8925 (14.7352, 333.375) -> (9.236, 323.85)
  line L8926 (9.236, 323.85) -> (14.7352, 314.325)
  line L8927 (14.7352, 314.325) -> (25.7337, 314.325)
  line L8928 (31.233, 323.85) -> (25.7337, 333.375)
  line L8929 (25.7337, 314.325) -> (31.233, 323.85)
  line L8930 (44.9812, 344.4875) -> (33.9826, 344.4875)
  line L8931 (33.9826, 344.4875) -> (28.4834, 334.9625)
  line L8932 (28.4834, 334.9625) -> (33.9826, 325.4375)
  line L8933 (33.9826, 325.4375) -> (44.9812, 325.4375)
  line L8934 (50.4804, 334.9625) -> (44.9812, 344.4875)
  line L8935 (44.9812, 325.4375) -> (50.4804, 334.9625)
  line L8936 (64.2286, 355.6) -> (53.2301, 355.6)
  line L8937 (53.2301, 355.6) -> (47.7308, 346.075)
  line L8938 (47.7308, 346.075) -> (53.2301, 336.55)
  line L8939 (53.2301, 336.55) -> (64.2286, 336.55)
  line L8940 (69.7278, 346.075) -> (64.2286, 355.6)
  line L8941 (64.2286, 336.55) -> (69.7278, 346.075)
  line L8942 (83.476, 366.7125) -> (72.4775, 366.7125)
  line L8943 (72.4775, 366.7125) -> (66.9782, 357.1875)
  line L8944 (66.9782, 357.1875) -> (72.4775, 347.6625)
  line L8945 (72.4775, 347.6625) -> (83.476, 347.6625)
  line L8946 (88.9753, 357.1875) -> (83.476, 366.7125)
  line L8947 (83.476, 347.6625) -> (88.9753, 357.1875)
  line L8948 (102.7234, 377.825) -> (91.7249, 377.825)
  line L8949 (91.7249, 377.825) -> (86.2256, 368.3)
  line L8950 (86.2256, 368.3) -> (91.7249, 358.775)
  line L8951 (91.7249, 358.775) -> (102.7234, 358.775)
  line L8952 (108.2227, 368.3) -> (102.7234, 377.825)
  line L8953 (102.7234, 358.775) -> (108.2227, 368.3)
  line L8954 (121.9708, 388.9375) -> (110.9723, 388.9375)
  line L8955 (110.9723, 388.9375) -> (105.473, 379.4125)
  line L8956 (105.473, 379.4125) -> (110.9723, 369.8875)
  line L8957 (110.9723, 369.8875) -> (121.9708, 369.8875)
  line L8958 (127.4701, 379.4125) -> (121.9708, 388.9375)
  line L8959 (121.9708, 369.8875) -> (127.4701, 379.4125)
  line L8960 (141.2182, 400.05) -> (130.2197, 400.05)
  line L8961 (130.2197, 400.05) -> (124.7205, 390.525)
  line L8962 (124.7205, 390.525) -> (130.2197, 381)
  line L8963 (130.2197, 381) -> (141.2182, 381)
  line L8964 (146.7175, 390.525) -> (141.2182, 400.05)
  line L8965 (141.2182, 381) -> (146.7175, 390.525)
  line L8966 (160.4657, 411.1625) -> (149.4671, 411.1625)
  line L8967 (149.4671, 411.1625) -> (143.9679, 401.6375)
  line L8968 (143.9679, 401.6375) -> (149.4671, 392.1125)
  line L8969 (149.4671, 392.1125) -> (160.4657, 392.1125)
  line L8970 (165.9649, 401.6375) -> (160.4657, 411.1625)
  line L8971 (160.4657, 392.1125) -> (165.9649, 401.6375)
  line L8972 (179.7131, 422.275) -> (168.7145, 422.275)
  line L8973 (168.7145, 422.275) -> (163.2153, 412.75)
  line L8974 (163.2153, 412.75) -> (168.7145, 403.225)
  line L8975 (168.7145, 403.225) -> (179.7131, 403.225)
  line L8976 (185.2123, 412.75) -> (179.7131, 422.275)
  line L8977 (179.7131, 403.225) -> (185.2123, 412.75)
  line L8978 (198.9605, 433.3875) -> (187.962, 433.3875)
  line L8979 (187.962, 433.3875) -> (182.4627, 423.8625)
  line L8980 (182.4627, 423.8625) -> (187.962, 414.3375)
  line L8981 (187.962, 414.3375) -> (198.9605, 414.3375)
  line L8982 (204.4597, 423.8625) -> (198.9605, 433.3875)
  line L8983 (198.9605, 414.3375) -> (204.4597, 423.8625)
  line L8984 (218.2079, 444.5) -> (207.2094, 444.5)
  line L8985 (207.2094, 444.5) -> (201.7101, 434.975)
  line L8986 (201.7101, 434.975) -> (207.2094, 425.45)
  line L8987 (207.2094, 425.45) -> (218.2079, 425.45)
  line L8988 (223.7072, 434.975) -> (218.2079, 444.5)
  line L8989 (218.2079, 425.45) -> (223.7072, 434.975)
  line L8990 (237.4553, 455.6125) -> (226.4568, 455.6125)
  line L8991 (226.4568, 455.6125) -> (220.9575, 446.0875)
  line L8992 (220.9575, 446.0875) -> (226.4568, 436.5625)
  line L8993 (226.4568, 436.5625) -> (237.4553, 436.5625)
  line L8994 (242.9546, 446.0875) -> (237.4553, 455.6125)
  line L8995 (237.4553, 436.5625) -> (242.9546, 446.0875)
  line L8996 (256.7027, 466.725) -> (245.7042, 466.725)
  line L8997 (245.7042, 466.725) -> (240.2049, 457.2)
  line L8998 (240.2049, 457.2) -> (245.7042, 447.675)
  line L8999 (245.7042, 447.675) -> (256.7027, 447.675)
  line L9000 (262.202, 457.2) -> (256.7027, 466.725)
  line L9001 (256.7027, 447.675) -> (262.202, 457.2)
  line L9002 (275.9501, 477.8375) -> (264.9516, 477.8375)
  line L9003 (264.9516, 477.8375) -> (259.4524, 468.3125)
  line L9004 (259.4524, 468.3125) -> (264.9516, 458.7875)
  line L9005 (264.9516, 458.7875) -> (275.9501, 458.7875)
  line L9006 (281.4494, 468.3125) -> (275.9501, 477.8375)
  line L9007 (275.9501, 458.7875) -> (281.4494, 468.3125)
  line L9008 (295.1976, 488.95) -> (284.199, 488.95)
  line L9009 (284.199, 488.95) -> (278.6998, 479.425)
  line L9010 (278.6998, 479.425) -> (284.199, 469.9)
  line L9011 (284.199, 469.9) -> (295.1976, 469.9)
  line L9012 (300.6968, 479.425) -> (295.1976, 488.95)
  line L9013 (295.1976, 469.9) -> (300.6968, 479.425)
  line L9014 (-859.6473, -155.575) -> (-870.6458, -155.575)
  line L9015 (-870.6458, -155.575) -> (-876.1451, -165.1)
  line L9016 (-876.1451, -165.1) -> (-870.6458, -174.625)
  line L9017 (-870.6458, -174.625) -> (-859.6473, -174.625)
  line L9018 (-854.1481, -165.1) -> (-859.6473, -155.575)
  line L9019 (-859.6473, -174.625) -> (-854.1481, -165.1)
  line L9020 (-840.3999, -144.4625) -> (-851.3984, -144.4625)
  line L9021 (-851.3984, -144.4625) -> (-856.8977, -153.9875)
  line L9022 (-856.8977, -153.9875) -> (-851.3984, -163.5125)
  line L9023 (-851.3984, -163.5125) -> (-840.3999, -163.5125)
  line L9024 (-834.9006, -153.9875) -> (-840.3999, -144.4625)
  line L9025 (-840.3999, -163.5125) -> (-834.9006, -153.9875)
  line L9026 (-821.1525, -133.35) -> (-832.151, -133.35)
  line L9027 (-832.151, -133.35) -> (-837.6503, -142.875)
  line L9028 (-837.6503, -142.875) -> (-832.151, -152.4)
  line L9029 (-832.151, -152.4) -> (-821.1525, -152.4)
  line L9030 (-815.6532, -142.875) -> (-821.1525, -133.35)
  line L9031 (-821.1525, -152.4) -> (-815.6532, -142.875)
  line L9032 (-801.9051, -122.2375) -> (-812.9036, -122.2375)
  line L9033 (-812.9036, -122.2375) -> (-818.4029, -131.7625)
  line L9034 (-818.4029, -131.7625) -> (-812.9036, -141.2875)
  line L9035 (-812.9036, -141.2875) -> (-801.9051, -141.2875)
  line L9036 (-796.4058, -131.7625) -> (-801.9051, -122.2375)
  line L9037 (-801.9051, -141.2875) -> (-796.4058, -131.7625)
  line L9038 (-782.6577, -111.125) -> (-793.6562, -111.125)
  line L9039 (-793.6562, -111.125) -> (-799.1554, -120.65)
  line L9040 (-799.1554, -120.65) -> (-793.6562, -130.175)
  line L9041 (-793.6562, -130.175) -> (-782.6577, -130.175)
  line L9042 (-777.1584, -120.65) -> (-782.6577, -111.125)
  line L9043 (-782.6577, -130.175) -> (-777.1584, -120.65)
  line L9044 (-763.4102, -100.0125) -> (-774.4088, -100.0125)
  line L9045 (-774.4088, -100.0125) -> (-779.908, -109.5375)
  line L9046 (-779.908, -109.5375) -> (-774.4088, -119.0625)
  line L9047 (-774.4088, -119.0625) -> (-763.4102, -119.0625)
  line L9048 (-757.911, -109.5375) -> (-763.4102, -100.0125)
  line L9049 (-763.4102, -119.0625) -> (-757.911, -109.5375)
  line L9050 (-744.1628, -88.9) -> (-755.1614, -88.9)
  line L9051 (-755.1614, -88.9) -> (-760.6606, -98.425)
  line L9052 (-760.6606, -98.425) -> (-755.1614, -107.95)
  line L9053 (-755.1614, -107.95) -> (-744.1628, -107.95)
  line L9054 (-738.6636, -98.425) -> (-744.1628, -88.9)
  line L9055 (-744.1628, -107.95) -> (-738.6636, -98.425)
  line L9056 (-724.9154, -77.7875) -> (-735.9139, -77.7875)
  line L9057 (-735.9139, -77.7875) -> (-741.4132, -87.3125)
  line L9058 (-741.4132, -87.3125) -> (-735.9139, -96.8375)
  line L9059 (-735.9139, -96.8375) -> (-724.9154, -96.8375)
  line L9060 (-719.4162, -87.3125) -> (-724.9154, -77.7875)
  line L9061 (-724.9154, -96.8375) -> (-719.4162, -87.3125)
  line L9062 (-705.668, -66.675) -> (-716.6665, -66.675)
  line L9063 (-716.6665, -66.675) -> (-722.1658, -76.2)
  line L9064 (-722.1658, -76.2) -> (-716.6665, -85.725)
  line L9065 (-716.6665, -85.725) -> (-705.668, -85.725)
  line L9066 (-700.1687, -76.2) -> (-705.668, -66.675)
  line L9067 (-705.668, -85.725) -> (-700.1687, -76.2)
  line L9068 (-686.4206, -55.5625) -> (-697.4191, -55.5625)
  line L9069 (-697.4191, -55.5625) -> (-702.9184, -65.0875)
  line L9070 (-702.9184, -65.0875) -> (-697.4191, -74.6125)
  line L9071 (-697.4191, -74.6125) -> (-686.4206, -74.6125)
  line L9072 (-680.9213, -65.0875) -> (-686.4206, -55.5625)
  line L9073 (-686.4206, -74.6125) -> (-680.9213, -65.0875)
  line L9074 (-667.1732, -44.45) -> (-678.1717, -44.45)
  line L9075 (-678.1717, -44.45) -> (-683.671, -53.975)
  line L9076 (-683.671, -53.975) -> (-678.1717, -63.5)
  line L9077 (-678.1717, -63.5) -> (-667.1732, -63.5)
  line L9078 (-661.6739, -53.975) -> (-667.1732, -44.45)
  line L9079 (-667.1732, -63.5) -> (-661.6739, -53.975)
  line L9080 (-647.9258, -33.3375) -> (-658.9243, -33.3375)
  line L9081 (-658.9243, -33.3375) -> (-664.4235, -42.8625)
  line L9082 (-664.4235, -42.8625) -> (-658.9243, -52.3875)
  line L9083 (-658.9243, -52.3875) -> (-647.9258, -52.3875)
  line L9084 (-642.4265, -42.8625) -> (-647.9258, -33.3375)
  line L9085 (-647.9258, -52.3875) -> (-642.4265, -42.8625)
  line L9086 (-628.6783, -22.225) -> (-639.6769, -22.225)
  line L9087 (-639.6769, -22.225) -> (-645.1761, -31.75)
  line L9088 (-645.1761, -31.75) -> (-639.6769, -41.275)
  line L9089 (-639.6769, -41.275) -> (-628.6783, -41.275)
  line L9090 (-623.1791, -31.75) -> (-628.6783, -22.225)
  line L9091 (-628.6783, -41.275) -> (-623.1791, -31.75)
  line L9092 (-609.4309, -11.1125) -> (-620.4295, -11.1125)
  line L9093 (-620.4295, -11.1125) -> (-625.9287, -20.6375)
  line L9094 (-625.9287, -20.6375) -> (-620.4295, -30.1625)
  line L9095 (-620.4295, -30.1625) -> (-609.4309, -30.1625)
  line L9096 (-603.9317, -20.6375) -> (-609.4309, -11.1125)
  line L9097 (-609.4309, -30.1625) -> (-603.9317, -20.6375)
  line L9098 (-590.1835, 0) -> (-601.182, 0)
  line L9099 (-601.182, 0) -> (-606.6813, -9.525)
  line L9100 (-606.6813, -9.525) -> (-601.182, -19.05)
  line L9101 (-601.182, -19.05) -> (-590.1835, -19.05)
  line L9102 (-584.6843, -9.525) -> (-590.1835, 0)
  line L9103 (-590.1835, -19.05) -> (-584.6843, -9.525)
  line L9104 (-570.9361, 11.1125) -> (-581.9346, 11.1125)
  line L9105 (-581.9346, 11.1125) -> (-587.4339, 1.5875)
  line L9106 (-587.4339, 1.5875) -> (-581.9346, -7.9375)
  line L9107 (-581.9346, -7.9375) -> (-570.9361, -7.9375)
  line L9108 (-565.4368, 1.5875) -> (-570.9361, 11.1125)
  line L9109 (-570.9361, -7.9375) -> (-565.4368, 1.5875)
  line L9110 (-551.6887, 22.225) -> (-562.6872, 22.225)
  line L9111 (-562.6872, 22.225) -> (-568.1865, 12.7)
  line L9112 (-568.1865, 12.7) -> (-562.6872, 3.175)
  line L9113 (-562.6872, 3.175) -> (-551.6887, 3.175)
  line L9114 (-546.1894, 12.7) -> (-551.6887, 22.225)
  line L9115 (-551.6887, 3.175) -> (-546.1894, 12.7)
  line L9116 (-532.4413, 33.3375) -> (-543.4398, 33.3375)
  line L9117 (-543.4398, 33.3375) -> (-548.9391, 23.8125)
  line L9118 (-548.9391, 23.8125) -> (-543.4398, 14.2875)
  line L9119 (-543.4398, 14.2875) -> (-532.4413, 14.2875)
  line L9120 (-526.942, 23.8125) -> (-532.4413, 33.3375)
  line L9121 (-532.4413, 14.2875) -> (-526.942, 23.8125)
  line L9122 (-513.1939, 44.45) -> (-524.1924, 44.45)
  line L9123 (-524.1924, 44.45) -> (-529.6916, 34.925)
  line L9124 (-529.6916, 34.925) -> (-524.1924, 25.4)
  line L9125 (-524.1924, 25.4) -> (-513.1939, 25.4)
  line L9126 (-507.6946, 34.925) -> (-513.1939, 44.45)
  line L9127 (-513.1939, 25.4) -> (-507.6946, 34.925)
  line L9128 (-493.9464, 55.5625) -> (-504.945, 55.5625)
  line L9129 (-504.945, 55.5625) -> (-510.4442, 46.0375)
  line L9130 (-510.4442, 46.0375) -> (-504.945, 36.5125)
  line L9131 (-504.945, 36.5125) -> (-493.9464, 36.5125)
  line L9132 (-488.4472, 46.0375) -> (-493.9464, 55.5625)
  line L9133 (-493.9464, 36.5125) -> (-488.4472, 46.0375)
  line L9134 (-474.699, 66.675) -> (-485.6976, 66.675)
  line L9135 (-485.6976, 66.675) -> (-491.1968, 57.15)
  line L9136 (-491.1968, 57.15) -> (-485.6976, 47.625)
  line L9137 (-485.6976, 47.625) -> (-474.699, 47.625)
  line L9138 (-469.1998, 57.15) -> (-474.699, 66.675)
  line L9139 (-474.699, 47.625) -> (-469.1998, 57.15)